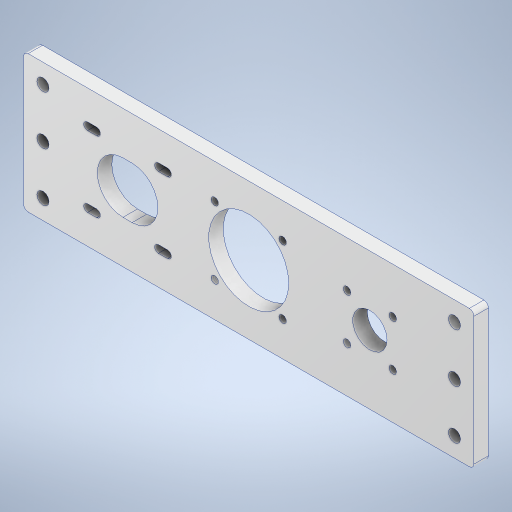
# Autodesk Inventor part: Z-Axis Drive Mount RevII
Saved by Autodesk Inventor 2024 (Build 280153000, 153)
## iProperties
Created: 2024-12-31
Part Number: Z-Axis Drive Mount RevII
Material: Aluminum 6061
Document SubType Name: Modeling
Designer: Ishaan
Density: 2.7 g/cm^3
Appearance: Aluminum - Flat
Author: Ishaan
Autodesk Inventor part; units mm, degrees
ref_plane "YZ Plane" through (0, 0, 0) normal (1, 0, 0) x (0, 1, 0)
ref_plane "XZ Plane" through (0, 0, 0) normal (0, 1, 0) x (-1, 0, 0)
ref_plane "XY Plane" through (0, 0, 0) normal (0, 0, 1) x (1, 0, 0)
sketch "Sketch1" plane through (0, 0, 0) normal (0, 0, 1) x (1, 0, 0)
  circle A0 centre (0, 0) radius 17.5
  line L0 (14.8492, -14.8492) -> (-14.8492, -14.8492) construction
  line L1 (-14.8492, -14.8492) -> (-14.8492, 14.8492) construction
  line L2 (-14.8492, 14.8492) -> (14.8492, 14.8492) construction
  line L3 (14.8492, 14.8492) -> (14.8492, -14.8492) construction
  line L4 (14.8492, -14.8492) -> (-14.8492, 14.8492) construction
  line L5 (-14.8492, -14.8492) -> (14.8492, 14.8492) construction
  circle A1 centre (0, 0) radius 21 construction
  line L6 (21, -21) -> (-21, -21) construction
  line L7 (-21, -21) -> (-21, 21) construction
  line L8 (-21, 21) -> (21, 21) construction
  line L9 (21, 21) -> (21, -21) construction
  line L10 (21, -21) -> (-21, 21) construction
  line L11 (-21, -21) -> (21, 21) construction
  line L12 (-31.85, -21.15) -> (-74.15, -21.15) construction
  line L13 (-74.15, -21.15) -> (-74.15, 21.15) construction
  line L14 (-74.15, 21.15) -> (-31.85, 21.15) construction
  line L15 (-31.85, 21.15) -> (-31.85, -21.15) construction
  line L16 (-31.85, -21.15) -> (-74.15, 21.15) construction
  line L17 (-74.15, -21.15) -> (-31.85, 21.15) construction
  line L18 (-37.5, -15.5) -> (-68.5, -15.5) construction
  line L19 (-68.5, -15.5) -> (-68.5, 15.5) construction
  line L20 (-68.5, 15.5) -> (-37.5, 15.5) construction
  line L21 (-37.5, 15.5) -> (-37.5, -15.5) construction
  line L22 (-37.5, -15.5) -> (-68.5, 15.5) construction
  line L23 (-68.5, -15.5) -> (-37.5, 15.5) construction
  line L24 (-70.5, 15.5) -> (-66.5, 15.5) construction
  line L25 (-70.5, 13.85) -> (-66.5, 13.85)
  line L26 (-66.5, 17.15) -> (-70.5, 17.15)
  arc A2 (-70.5, 17.15) -> (-70.5, 13.85) centre (-70.5, 15.5) ccw
  arc A3 (-66.5, 13.85) -> (-66.5, 17.15) centre (-66.5, 15.5) ccw
  line L27 (-35.5, 15.5) -> (-39.5, 15.5) construction
  line L28 (-35.5, 17.15) -> (-39.5, 17.15)
  line L29 (-39.5, 13.85) -> (-35.5, 13.85)
  arc A4 (-35.5, 13.85) -> (-35.5, 17.15) centre (-35.5, 15.5) ccw
  arc A5 (-39.5, 17.15) -> (-39.5, 13.85) centre (-39.5, 15.5) ccw
  line L30 (-35.5, -15.5) -> (-39.5, -15.5) construction
  line L31 (-35.5, -13.85) -> (-39.5, -13.85)
  line L32 (-39.5, -17.15) -> (-35.5, -17.15)
  arc A6 (-35.5, -17.15) -> (-35.5, -13.85) centre (-35.5, -15.5) ccw
  arc A7 (-39.5, -13.85) -> (-39.5, -17.15) centre (-39.5, -15.5) ccw
  line L33 (-70.5, -15.5) -> (-66.5, -15.5) construction
  line L34 (-70.5, -17.15) -> (-66.5, -17.15)
  line L35 (-66.5, -13.85) -> (-70.5, -13.85)
  arc A8 (-70.5, -13.85) -> (-70.5, -17.15) centre (-70.5, -15.5) ccw
  arc A9 (-66.5, -17.15) -> (-66.5, -13.85) centre (-66.5, -15.5) ccw
  line L36 (-55, 0) -> (-51, 0) construction
  line L37 (-55, -11.25) -> (-51, -11.25)
  line L38 (-51, 11.25) -> (-55, 11.25)
  arc A10 (-55, 11.25) -> (-55, -11.25) centre (-55, 0) ccw
  arc A11 (-51, -11.25) -> (-51, 11.25) centre (-51, 0) ccw
  line L39 (40, 54.25) -> (-40, 54.25) construction
  line L40 (-40, 54.25) -> (-40, 94.25) construction
  line L41 (-40, 94.25) -> (40, 94.25) construction
  line L42 (40, 94.25) -> (40, 54.25) construction
  line L43 (40, 54.25) -> (-40, 94.25) construction
  line L44 (-40, 54.25) -> (40, 94.25) construction
  line L45 (98.5, -30) -> (-98.5, -30)
  line L46 (-98.5, -30) -> (-98.5, 30)
  line L47 (-98.5, 30) -> (98.5, 30)
  line L48 (98.5, 30) -> (98.5, -30)
  line L49 (98.5, -30) -> (-98.5, 30) construction
  line L50 (-98.5, -30) -> (98.5, 30) construction
  line L51 (-77, 22) -> (-29, 22)
  line L52 (-29, 22) -> (-29, -22)
  line L53 (-29, -22) -> (-77, -22)
  line L54 (-77, -22) -> (-77, 22)
  line L55 (-77, 22) -> (-29, -22) construction
  line L56 (-29, 22) -> (-77, -22) construction
  line L57 (80, 30) -> (100, 30) construction
  line L58 (100, 30) -> (100, -30) construction
  line L59 (100, -30) -> (80, -30) construction
  line L60 (80, -30) -> (80, 30) construction
  line L61 (80, 30) -> (100, -30) construction
  line L62 (100, 30) -> (80, -30) construction
  line L63 (-80, 30) -> (-100, 30) construction
  line L64 (-100, 30) -> (-100, -30) construction
  line L65 (-100, -30) -> (-80, -30) construction
  line L66 (-80, -30) -> (-80, 30) construction
  line L67 (-80, 30) -> (-100, -30) construction
  line L68 (-100, 30) -> (-80, -30) construction
  line L69 (-83, -28) -> (-23, -28) construction
  line L70 (-23, -28) -> (-23, 28) construction
  line L71 (-23, 28) -> (-83, 28) construction
  line L72 (-83, 28) -> (-83, -28) construction
  circle A12 centre (0, 0) radius 34 construction
  line L73 (-28, -28) -> (28, -28) construction
  line L74 (28, -28) -> (28, 28) construction
  line L75 (28, 28) -> (-28, 28) construction
  line L76 (-28, 28) -> (-28, -28) construction
  line L77 (-28, -28) -> (28, 28) construction
  line L78 (28, -28) -> (-28, 28) construction
  circle A13 centre (0, 0) radius 25 construction
  line L79 (0, 0) -> (9.5671, 23.097) construction
  point P0 (-53, 0)
  point P1 (0, 74.25)
  point P2 (90, 0)
  point P3 (-90, 0)
  dimension "d1" = 42
  dimension "d44" = 50
  dimension "d0" = 35
  dimension "d2" = 42
  dimension "d3" = 42
  dimension "d4" = 42.3
  dimension "d5" = 42.3
  dimension "d6" = 53
  dimension "d7" = 31
  dimension "d8" = 31
  dimension "d9" = 1.65
  dimension "d10" = 4
  dimension "d11" = 11.25
  dimension "d12" = 80
  dimension "d13" = 40
  dimension "d14" = 54.25
  dimension "d15" = 197
  dimension "d16" = 60
  dimension "d35" = 48
  dimension "d36" = 44
  dimension "d37" = 20
  dimension "d38" = 90
  dimension "d39" = 90
  dimension "d40" = 6
  dimension "d41" = 68
  dimension "d42" = 56
  dimension "d43" = 56
  dimension "d45" = 22.5
  constraints: 170 end point, 27 parallel, 25 midpoint, 20 point on circle, 20 tangent, 12 centre point, 11 horizontal, 11 perpendicular, 8 coincident, 6 equal length, 5 point on line, 3 collinear, 3 equal radius, 1 horizontal alignment, 1 vertical alignment, 9 other
  measures "d0" diameter of A0
  measures "d2" distance of L7.end L8.end
  measures "d3" distance of L6.end L7.end
  measures "d4" distance of L13.end L14.end
  measures "d5" distance of L12.end L13.end
  measures "d6" distance of point (0, 0) point (-53, 0)
  measures "d7" distance of L19.end L20.end
  measures "d8" distance of L18.end L19.end
  measures "d9" radius of A3
  measures "d10" distance of L26.start L26.end
  measures "d11" radius of A11
  measures "d12" distance of L40.end L41.end
  measures "d13" distance of L39.end L40.end
  measures "d14" distance from line of point (0, 0) L39
  measures "d15" distance of L46.end L47.end
  measures "d16" distance of L45.end L46.end
  measures "d35" distance of L52.end L53.end
  measures "d36" distance of L51.end L52.end
  measures "d37" distance of L58.end L59.end
  measures "d38" distance of point (0, 0) point (90, 0)
  measures "d39" distance of point (0, 0) point (-90, 0)
  measures "d40" distance between parallel lines of L53 L69
  measures "d41" diameter of A12
  measures "d42" distance of L75.end L74.end
  measures "d43" distance of L74.end L73.end
  measures "d45" angle of L74 L79
extrude "Extrusion1" add sketch "Sketch1" along normal blind 6.35 contours L45 L46 L47 L48 | L51 L52 L53 L54
hole "Hole3" at (14.8492, 14.8492, 0) at (-14.8492, 14.8492, 0) at (14.8492, -14.8492, 0) at (-14.8492, -14.8492, 0) direction (0, 0, 1) diameter 3.242 end through all thread size "M4x0.7" class "6H" standard "ANSI Metric M Profile"
sketch "Sketch2" plane through (0, 0, 6.35) normal (0, 0, 1) x (1, 0, 0)
  line L0 (90, -21.5) -> (-90, -21.5) construction
  line L1 (-90, -21.5) -> (-90, 21.5) construction
  line L2 (-90, 21.5) -> (90, 21.5) construction
  line L3 (90, 21.5) -> (90, -21.5) construction
  line L4 (90, -21.5) -> (-90, 21.5) construction
  line L5 (-90, -21.5) -> (90, 21.5) construction
  line L6 (98.5, 30) -> (-98.5, 30) construction
  line L7 (-98.5, 30) -> (-90, 30) construction
  line L8 (-90, 30) -> (-90, 21.5) construction
  line L9 (-90, 21.5) -> (-98.5, 21.5) construction
  line L10 (-98.5, 21.5) -> (-98.5, 30) construction
  point P0 (0, 0)
  point P1 (-90, 0)
  point P2 (90, 0)
  dimension "d26" = 180
  constraints: 20 end point, 4 coincident, 4 midpoint, 4 parallel, 3 perpendicular, 2 horizontal
  measures "d26" distance of L0.start L0.end
hole "Hole2" at (-90, 0, 6.35) at (-90, 21.5, 6.35) at (-90, -21.5, 6.35) at (90, 21.5, 6.35) at (90, 0, 6.35) at (90, -21.5, 6.35) direction (0, 0, -1) diameter 5.3 end through all
fillet "Fillet1" radius 2 4 edges at (-98.5, -30, 3.175) (-98.5, 30, 3.175) (98.5, 30, 3.175) (98.5, -30, 3.175)
sketch "Sketch3" plane through (0, 0, 0) normal (0, 0, -1) x (-1, 0, 0)
  line L0 (53, 0) -> (-53, 0) construction
  line L1 (-43, -10) -> (-63, -10) construction
  line L2 (-63, -10) -> (-63, 10) construction
  line L3 (-63, 10) -> (-43, 10) construction
  line L4 (-43, 10) -> (-43, -10) construction
  line L5 (-43, -10) -> (-63, 10) construction
  line L6 (-63, -10) -> (-43, 10) construction
  circle A0 centre (-53, 0) radius 7.5
  point P0 (0, 0)
  point P1 (0, 0)
  dimension "d56" = 20
  dimension "d57" = 20
  dimension "d58" = 15
  constraints: 14 end point, 6 coincident, 3 midpoint, 2 parallel, 1 centre point, 1 horizontal, 1 perpendicular
  measures "d56" distance of L2.end L3.end
  measures "d57" distance of L1.end L2.end
  measures "d58" diameter of A0
extrude "Extrusion2" cut sketch "Sketch3" against normal through all
hole "Hole4" at (-53, 0, 0) at (63, 10, 0) at (43, 10, 0) at (43, -10, 0) at (63, -10, 0) direction (0, 0, 1) diameter 3.3 end through all
equation "\"d35\" = d36 + d10"
equation "\"d39\" = d38"
body "Solid1"
